Autodesk Inventor part; units mm, degrees
(part 2 of 2)
  spline S23 degree 2 poles (-11.6726, 3.9757) (-12.1172, 4.2968) (-12.5783, 5.2272) (-12.5783, 5.8529) knots 0 0 0 1 2 2 2
  spline S24 degree 2 poles (-12.5783, 5.8529) (-12.5783, 6.6927) (-11.475, 7.9607) (-10.7011, 8.1254) knots 0 0 0 1 2 2 2
  line L267 (-10.7011, 8.1254) -> (-10.7011, 8.2242)
  spline S25 degree 2 poles (-10.7011, 8.2242) (-11.0222, 8.29) (-11.755, 8.5864) (-12.0678, 8.8828) knots 0 0 0 1 2 2 2
  spline S26 degree 2 poles (-12.0678, 8.8828) (-12.3807, 9.171) (-12.7759, 10.0931) (-12.7759, 10.76) knots 0 0 0 1 2 2 2
  spline S27 degree 2 poles (-12.7759, 10.76) (-12.7759, 11.4434) (-12.3066, 12.6043) (-11.8785, 13.0489) knots 0 0 0 1 2 2 2
  spline S28 degree 2 poles (-11.8785, 13.0489) (-11.4339, 13.51) (-10.1742, 13.9875) (-9.3755, 13.9875) knots 0 0 0 1 2 2 2
  spline S29 degree 2 poles (-9.3755, 13.9875) (-8.6098, 13.9875) (-7.1113, 13.617) (-6.6009, 13.3618) knots 0 0 0 1 2 2 2
  line L268 (-6.6009, 13.3618) -> (-6.6009, 11.921)
  line L269 (-6.6009, 11.921) -> (-6.6997, 11.921)
  spline S30 degree 2 poles (-6.6997, 11.921) (-7.1278, 12.2338) (-8.5769, 12.8102) (-9.2932, 12.8102) knots 0 0 0 1 2 2 2
  spline S31 degree 2 poles (-9.2932, 12.8102) (-9.7131, 12.8102) (-10.5529, 12.5467) (-10.8328, 12.2421) knots 0 0 0 1 2 2 2
  spline S32 degree 2 poles (-10.8328, 12.2421) (-11.1045, 11.9374) (-11.3927, 11.2129) (-11.3927, 10.6612) knots 0 0 0 1 2 2 2
  spline S33 degree 2 poles (-11.3927, 10.6612) (-11.3927, 10.1096) (-11.0716, 9.3933) (-10.7834, 9.1875) knots 0 0 0 1 2 2 2
  spline S34 degree 2 poles (-10.7834, 9.1875) (-10.4953, 8.9816) (-9.7131, 8.8252) (-9.252, 8.8252) knots 0 0 0 1 2 2 2
  line L270 (-9.252, 8.8252) -> (-8.6757, 8.8252)
  line L271 (-8.6757, 8.8252) -> (-8.6757, 7.6972)
  line L272 (-8.6757, 7.6972) -> (-9.1285, 7.6972)
  spline S35 degree 2 poles (-9.1285, 7.6972) (-10.0424, 7.6972) (-11.1951, 6.8245) (-11.1951, 5.9929) knots 0 0 0 1 2 2 2
  spline S36 degree 2 poles (-11.1951, 5.9929) (-11.1951, 5.6059) (-10.8987, 5.0543) (-10.6599, 4.8896) knots 0 0 0 1 2 2 2
  spline S37 degree 2 poles (-10.6599, 4.8896) (-10.4047, 4.7167) (-9.779, 4.5768) (-9.4249, 4.5768) knots 0 0 0 1 2 2 2
  spline S38 degree 2 poles (-9.4249, 4.5768) (-9.0544, 4.5768) (-8.3216, 4.7579) (-7.9676, 4.8979) knots 0 0 0 1 2 2 2
  spline S39 degree 2 poles (-7.9676, 4.8979) (-7.6383, 5.0378) (-7.1525, 5.3342) (-6.9631, 5.466) knots 0 0 0 1 2 2 2
  line L273 (-6.9631, 5.466) -> (-6.8808, 5.466)
  line L274 (-6.8808, 5.466) -> (-6.8808, 4.0251)
  spline S40 degree 2 poles (-6.8808, 4.0251) (-7.3254, 3.7864) (-8.8486, 3.3994) (-9.532, 3.3994) knots 0 0 0 1 2 2 2
  spline S41 degree 2 poles (-9.532, 3.3994) (-10.2236, 3.3994) (-11.2527, 3.6793) (-11.6726, 3.9757) knots 0 0 0 1 2 2 2
  spline S42 degree 2 poles (-11.6726, 3.9757) (-12.1172, 4.2968) (-12.5783, 5.2272) (-12.5783, 5.8529) knots 0 0 0 1 2 2 2
  spline S43 degree 2 poles (-12.5783, 5.8529) (-12.5783, 6.6927) (-11.475, 7.9607) (-10.7011, 8.1254) knots 0 0 0 1 2 2 2
  line L275 (-10.7011, 8.1254) -> (-10.7011, 8.2242)
  spline S44 degree 2 poles (-10.7011, 8.2242) (-11.0222, 8.29) (-11.755, 8.5864) (-12.0678, 8.8828) knots 0 0 0 1 2 2 2
  spline S45 degree 2 poles (-12.0678, 8.8828) (-12.3807, 9.171) (-12.7759, 10.0931) (-12.7759, 10.76) knots 0 0 0 1 2 2 2
  spline S46 degree 2 poles (-12.7759, 10.76) (-12.7759, 11.4434) (-12.3066, 12.6043) (-11.8785, 13.0489) knots 0 0 0 1 2 2 2
  spline S47 degree 2 poles (-11.8785, 13.0489) (-11.4339, 13.51) (-10.1742, 13.9875) (-9.3755, 13.9875) knots 0 0 0 1 2 2 2
  spline S48 degree 2 poles (-9.3755, 13.9875) (-8.6098, 13.9875) (-7.1113, 13.617) (-6.6009, 13.3618) knots 0 0 0 1 2 2 2
  line L276 (-6.6009, 13.3618) -> (-6.6009, 11.921)
  line L277 (-6.6009, 11.921) -> (-6.6997, 11.921)
  spline S49 degree 2 poles (-6.6997, 11.921) (-7.1278, 12.2338) (-8.5769, 12.8102) (-9.2932, 12.8102) knots 0 0 0 1 2 2 2
  spline S50 degree 2 poles (-9.2932, 12.8102) (-9.7131, 12.8102) (-10.5529, 12.5467) (-10.8328, 12.2421) knots 0 0 0 1 2 2 2
  spline S51 degree 2 poles (-10.8328, 12.2421) (-11.1045, 11.9374) (-11.3927, 11.2129) (-11.3927, 10.6612) knots 0 0 0 1 2 2 2
  spline S52 degree 2 poles (-11.3927, 10.6612) (-11.3927, 10.1096) (-11.0716, 9.3933) (-10.7834, 9.1875) knots 0 0 0 1 2 2 2
  spline S53 degree 2 poles (-10.7834, 9.1875) (-10.4953, 8.9816) (-9.7131, 8.8252) (-9.252, 8.8252) knots 0 0 0 1 2 2 2
  line L278 (-9.252, 8.8252) -> (-8.6757, 8.8252)
  line L279 (-8.6757, 8.8252) -> (-8.6757, 7.6972)
  line L280 (-8.6757, 7.6972) -> (-9.1285, 7.6972)
  spline S54 degree 2 poles (-9.1285, 7.6972) (-10.0424, 7.6972) (-11.1951, 6.8245) (-11.1951, 5.9929) knots 0 0 0 1 2 2 2
  spline S55 degree 2 poles (-11.1951, 5.9929) (-11.1951, 5.6059) (-10.8987, 5.0543) (-10.6599, 4.8896) knots 0 0 0 1 2 2 2
  spline S56 degree 2 poles (-10.6599, 4.8896) (-10.4047, 4.7167) (-9.779, 4.5768) (-9.4249, 4.5768) knots 0 0 0 1 2 2 2
  spline S57 degree 2 poles (-54.0751, 84.4929) (-54.4456, 84.4929) (-55.1784, 84.3117) (-55.5324, 84.1718) knots 0 0 0 1 2 2 2
  spline S58 degree 2 poles (-55.5324, 84.1718) (-55.8617, 84.0318) (-56.3475, 83.7354) (-56.5369, 83.6037) knots 0 0 0 1 2 2 2
  line L281 (-56.5369, 83.6037) -> (-56.6192, 83.6037)
  line L282 (-56.6192, 83.6037) -> (-56.6192, 85.0445)
  spline S59 degree 2 poles (-56.6192, 85.0445) (-56.1746, 85.2833) (-54.6514, 85.6702) (-53.968, 85.6702) knots 0 0 0 1 2 2 2
  spline S60 degree 2 poles (-53.968, 85.6702) (-53.2764, 85.6702) (-52.2473, 85.3903) (-51.8274, 85.0939) knots 0 0 0 1 2 2 2
  spline S61 degree 2 poles (-51.8274, 85.0939) (-51.3828, 84.7728) (-50.9217, 83.8424) (-50.9217, 83.2167) knots 0 0 0 1 2 2 2
  spline S62 degree 2 poles (-50.9217, 83.2167) (-50.9217, 82.3769) (-52.025, 81.1089) (-52.7989, 80.9443) knots 0 0 0 1 2 2 2
  line L283 (-52.7989, 80.9443) -> (-52.7989, 80.8455)
  spline S63 degree 2 poles (-52.7989, 80.8455) (-52.4778, 80.7796) (-51.745, 80.4832) (-51.4322, 80.1868) knots 0 0 0 1 2 2 2
  spline S64 degree 2 poles (-51.4322, 80.1868) (-51.1193, 79.8986) (-50.7241, 78.9765) (-50.7241, 78.3096) knots 0 0 0 1 2 2 2
  spline S65 degree 2 poles (-50.7241, 78.3096) (-50.7241, 77.6262) (-51.1934, 76.4653) (-51.6215, 76.0207) knots 0 0 0 1 2 2 2
  spline S66 degree 2 poles (-51.6215, 76.0207) (-52.0661, 75.5596) (-53.3258, 75.0821) (-54.1245, 75.0821) knots 0 0 0 1 2 2 2
  spline S67 degree 2 poles (-54.1245, 75.0821) (-54.8902, 75.0821) (-56.3887, 75.4526) (-56.8991, 75.7078) knots 0 0 0 1 2 2 2
  line L284 (-56.8991, 75.7078) -> (-56.8991, 77.1487)
  line L285 (-56.8991, 77.1487) -> (-56.8003, 77.1487)
  spline S68 degree 2 poles (-56.8003, 77.1487) (-56.3722, 76.8358) (-54.9231, 76.2595) (-54.2068, 76.2595) knots 0 0 0 1 2 2 2
  spline S69 degree 2 poles (-54.2068, 76.2595) (-53.7869, 76.2595) (-52.9471, 76.523) (-52.6672, 76.8276) knots 0 0 0 1 2 2 2
  spline S70 degree 2 poles (-52.6672, 76.8276) (-52.3955, 77.1322) (-52.1073, 77.8568) (-52.1073, 78.4084) knots 0 0 0 1 2 2 2
  spline S71 degree 2 poles (-52.1073, 78.4084) (-52.1073, 78.96) (-52.4284, 79.6763) (-52.7166, 79.8822) knots 0 0 0 1 2 2 2
  spline S72 degree 2 poles (-52.7166, 79.8822) (-53.0047, 80.088) (-53.7869, 80.2444) (-54.248, 80.2444) knots 0 0 0 1 2 2 2
  line L286 (-54.248, 80.2444) -> (-54.8243, 80.2444)
  line L287 (-54.8243, 80.2444) -> (-54.8243, 81.3724)
  line L288 (-54.8243, 81.3724) -> (-54.3715, 81.3724)
  spline S73 degree 2 poles (-54.3715, 81.3724) (-53.4576, 81.3724) (-52.3049, 82.2452) (-52.3049, 83.0767) knots 0 0 0 1 2 2 2
  spline S74 degree 2 poles (-52.3049, 83.0767) (-52.3049, 83.4637) (-52.6013, 84.0153) (-52.8401, 84.18) knots 0 0 0 1 2 2 2
  spline S75 degree 2 poles (-52.8401, 84.18) (-53.0953, 84.3529) (-53.721, 84.4929) (-54.0751, 84.4929) knots 0 0 0 1 2 2 2
  point P0 (-31.75, 44.45)
  point P1 (-31.75, 68.8958)
  point P2 (-31.75, 20.0009)
  point P3 (-53.7479, 68.8958)
  point P4 (-9.7521, 20.0042)
  point P5 (-41.8348, 101.4209)
  point P6 (-31.75, 68.8958)
  point P7 (-31.75, 44.45)
  point P8 (-31.75, 20.0009)
  point P9 (-53.7479, 68.8958)
  point P10 (-9.7521, 20.0042)
  point P11 (-1, 6.9835)
  dimension "d155" = 8.4153
  dimension "d157" = 0.508
  dimension "d158" = 4.5466
  dimension "d159" = 0.508
  dimension "d160" = 4.5466
  constraints: 488 end point, 50 parallel, 20 perpendicular, 14 horizontal, 1 midpoint, 14 other
  measures "d155" distance of L254.end L252.start
  measures "d157" distance between parallel lines of L7 L253
  measures "d158" distance from line of point (-1, 6.983) L252
  measures "d159" distance between parallel lines of L6 L248
  measures "d160" distance between parallel lines of L4 L251
extrude "Extrusion20" add sketch "Sketch17" along normal blind 0.4 contours L48 L49 L73 L71 L76 L69 L86 L79 L85 L67 L62 L68 L84 L80 L87 L77 L82 L60 L55 L61 L81 L78 L83 L70 L75 L72 L74 L50 | L88 L89 L113 L111 L116 L109 L126 L119 L125 L107 L102 L108 L124 L120 L127 L117 L122 L100 L95 L101 L121 L118 L123 L110 L115 L112 L114 L90 | L128 L129 L153 L151 L156 L149 L166 L159 L165 L147 L142 L148 L164 L160 L167 L157 L162 L140 L135 L141 L161 L158 L163 L150 L155 L152 L154 L130 | L168 L169 L193 L191 L196 L189 L206 L199 L205 L187 L182 L188 L204 L200 L207 L197 L202 L180 L175 L181 L201 L198 L203 L190 L195 L192 L194 L170 | L208 L209 L233 L231 L236 L229 L246 L239 L245 L227 L222 L228 L244 L240 L247 L237 L242 L220 L215 L221 L241 L238 L243 L230 L235 L232 L234 L210 | S0 S1 L257 L258 S2 S3 S4 S5 L259 S6 S7 S8 S9 S10 L260 L261 S11 S12 S13 S14 S15 L262 L263 L264 S16 S17 S18 | S19 S20 L265 L266 S21 S22 S23 S24 L267 S25 S26 S27 S28 S29 L268 L269 S30 S31 S32 S33 S34 L270 L271 L272 S35 S36 S37 bodies 2
sketch "Sketch18" plane through (0, 0, -0.2) normal (0, 0, -1) x (-1, 0, 0)
  line L0 (0, 0) -> (-63.5, 0)
  line L1 (-63.5, 0) -> (-63.5, 88.9)
  line L2 (-63.5, 88.9) -> (0, 88.9)
  line L3 (0, 88.9) -> (0, 0)
  constraints: 8 end point, 2 parallel, 1 horizontal, 1 perpendicular
extrude "Extrusion21" add sketch "Sketch18" along normal blind 0.4 bodies 3
fillet "Fillet2" radius 3.175 8 edges at (63.5, 0, 0.2) (63.5, 88.9, 0.2) (0, 0, 0.2) (0, 88.9, 0.2) (63.5, 0, -0.3) (63.5, 88.9, -0.3) (0, 0, -0.3) (0, 88.9, -0.3)
extrude "Extrusion22" cut sketch "Sketch17" along normal blind 0.4 contours L48 L49 L73 L71 L76 L69 L86 L79 L85 L67 L62 L68 L84 L80 L87 L77 L82 L60 L55 L61 L81 L78 L83 L70 L75 L72 L74 L50 | L88 L89 L113 L111 L116 L109 L126 L119 L125 L107 L102 L108 L124 L120 L127 L117 L122 L100 L95 L101 L121 L118 L123 L110 L115 L112 L114 L90 | L128 L129 L153 L151 L156 L149 L166 L159 L165 L147 L142 L148 L164 L160 L167 L157 L162 L140 L135 L141 L161 L158 L163 L150 L155 L152 L154 L130 | L168 L169 L193 L191 L196 L189 L206 L199 L205 L187 L182 L188 L204 L200 L207 L197 L202 L180 L175 L181 L201 L198 L203 L190 L195 L192 L194 L170 | L208 L209 L233 L231 L236 L229 L246 L239 L245 L227 L222 L228 L244 L240 L247 L237 L242 L220 L215 L221 L241 L238 L243 L230 L235 L232 L234 L210 | S0 S1 L257 L258 S2 S3 S4 S5 L259 S6 S7 S8 S9 S10 L260 L261 S11 S12 S13 S14 S15 L262 L263 L264 S16 S17 S18 | S19 S20 L265 L266 S21 S22 S23 S24 L267 S25 S26 S27 S28 S29 L268 L269 S30 S31 S32 S33 S34 L270 L271 L272 S35 S36 S37 bodies 3
